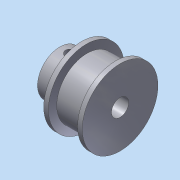
# Autodesk Inventor part: GT2 Timing Pulley
Saved by Autodesk Inventor 2013 (Build 170138000, 138)
## iProperties
Created: 2013-11-09
Part Number: GT2 Timing Pulley
Material: Aluminum 6061
Document SubType Name: Modeling
Designer: Jon Hollander
Density: 2.71 g/cm^3
Catalog Web Link: http://openbuildspartstore.com/gt2-2mm-aluminum-timing-pulley-30/
Description: GT2 (2mm) Aluminum Timing Pulley - 30
Mass: 9.67219 g
Surface Area: 22.068 cm^2
Volume: 3.56907 cm^3
Author: Jon Hollander
Autodesk Inventor part; units mm, degrees
note: some values were not read from the file. Chosen so that the rebuilt part matches the saved one: direction of "Hole2".
ref_plane "YZ Plane" through (0, 0, 0) normal (1, 0, 0) x (0, 1, 0)
ref_plane "XZ Plane" through (0, 0, 0) normal (0, 1, 0) x (-1, 0, 0)
sketch "Sketch1" plane through (0, 0, 0) normal (0, 0, 1) x (1, 0, 0)
  line L0 (0, 0) -> (17.5, 0)
  line L1 (0, 0) -> (0, 6.5)
  line L2 (0, 6.5) -> (6.3, 6.5)
  line L3 (6.3, 6.5) -> (6.3, 11)
  line L4 (6.3, 11) -> (7.658, 11)
  line L5 (7.658, 11) -> (7.9, 8.8125)
  line L6 (7.9, 8.8125) -> (15.9, 8.8125)
  line L7 (15.9, 8.8125) -> (16.142, 11)
  line L8 (16.142, 11) -> (17.5, 11)
  line L9 (17.5, 11) -> (17.5, 0)
  line L10 (7.658, 11) -> (16.142, 11) construction
  line L11 (11.9, 8.8125) -> (11.9, 11) construction
  dimension "d0" = 13
  dimension "d2" = 22
  dimension "d3" = 11.2
  dimension "d4" = 1.358
  dimension "d5" = 8
  dimension "d6" = 1.358
  dimension "d7" = 17.625
  dimension "d8" = 6.3
  dimension "d9" = 17.5
  constraints: 24 end point, 5 parallel, 3 perpendicular, 2 midpoint, 1 collinear, 1 horizontal, 1 vertical
  measures "d0" diameter of L2 L0
  measures "d2" diameter of L4 L0
  measures "d3" distance between parallel lines of L9 L3
  measures "d4" distance of L3.end L4.end
  measures "d5" distance of L5.end L6.end
  measures "d6" distance of L7.end L8.end
  measures "d7" diameter of L6 L0
  measures "d8" distance between parallel lines of L3 L1
  measures "d9" distance between parallel lines of L9 L1
revolve "Revolution1" add sketch "Sketch1" angle 360 about axis through (0, 0, 0) along (1, 0, 0)
sketch "Sketch2" plane through (17.5, 0, 0) normal (1, 0, 0) x (0, 0, -1)
  circle A0 centre (0, 0) radius 11 projected
  constraints: 1 coincident
hole "Hole1" at (17.5, 0, 0) direction (-1, 0, 0) diameter 5 end through all
ref_plane "Work Plane1" through (3.15, 0, 6.5) normal (0, 0, 1) x (1, 0, 0)
sketch "Sketch4" plane through (3.15, 0, 6.5) normal (0, 0, 1) x (1, 0, 0)
  line L0 (3.15, -6.5) -> (3.15, 6.5) projected
  line L1 (-3.15, -6.5) -> (-3.15, 6.5) projected
  line L2 (-3.15, 0) -> (3.15, 0) construction
  point P0 (0, 0)
  constraints: 2 end point, 2 midpoint
hole "Hole2" at (3.15, 0, 6.5) direction (0, 0, -1) diameter 3 end up to surface
pattern_circular "Circular Pattern1" count 2 over 90 about axis through (-18.1966, 0, 0) along (-1, 0, 0) of "Hole2"
equation "\"d6\" = d4"
body "Solid1"
